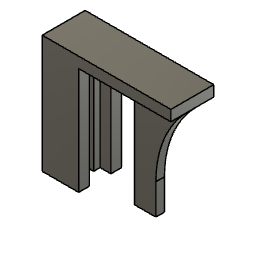
wall holder_ (Autodesk Fusion 360 design; units mm, degrees)
Autodesk Fusion 360 part; units mm, degrees
sketch "Esquisse1" plane through (0, 0, 0) normal (0, 1, 0) x (1, 0, 0)
  line L0 (-427, 120) -> (-367, 120)
  line L1 (-367, 120) -> (-367, 100)
  line L2 (-367, 100) -> (-427, 100)
  line L3 (-427, 100) -> (-427, 120)
  line L4 (-410, 120) -> (-410, 115)
  line L5 (-410, 115) -> (-415, 115)
  line L6 (-415, 115) -> (-415, 112)
  line L7 (-415, 112) -> (-417, 112)
  line L8 (-417, 112) -> (-417, 108)
  line L9 (-417, 108) -> (-415, 108)
  line L10 (-415, 105) -> (-415, 108)
  line L11 (-415, 105) -> (-410, 105)
  line L12 (-410, 100) -> (-410, 105)
  line L13 (-392, 112) -> (-382, 112)
  line L14 (-382, 112) -> (-382, 108)
  line L15 (-382, 108) -> (-392, 108)
  line L16 (-392, 108) -> (-392, 112)
  dimension "d5" = 20
  dimension "d6" = 60
  dimension "d7" = 5
  dimension "d8" = 3
  dimension "d9" = 5
  dimension "d10" = 2
  dimension "d12" = 4
  dimension "d13" = 3
  dimension "d14" = 2
  dimension "d15" = 5
  dimension "d16" = 5
  dimension "d17" = 10
  dimension "d18" = 4
  dimension "d19" = 25
  dimension "d26" = 10
  constraint horizontal L0
  constraint vertical L1
  constraint horizontal L2
  constraint vertical L3
  constraint coincident L0 L4.start
  constraint perpendicular L0 L4
  constraint perpendicular L4 L5
  constraint perpendicular L5 L6
  constraint perpendicular L6 L7
  constraint perpendicular L7 L8
  constraint perpendicular L8 L9
  constraint perpendicular L9 L10
  constraint perpendicular L10 L11
  constraint coincident L2 L12.start
  constraint perpendicular L11 L12
  constraint horizontal L13
  constraint vertical L14
  constraint horizontal L15
  constraint vertical L16
  measures "d5" distance of L0.end L1.end
  measures "d6" distance of L0.start L0.end
  measures "d7" distance of L4.start L4.end
  measures "d8" distance of L5.end L6.end
  measures "d9" distance of L4.end L5.end
  measures "d10" distance of L6.end L7.end
  measures "d12" distance of L7.end L8.end
  measures "d13" distance of L9.end L10.start
  measures "d14" distance of L8.end L9.end
  measures "d15" distance of L10.start L11.end
  measures "d16" distance of L11.end L12.start
  measures "d17" distance of L13.start L13.end
  measures "d18" distance of L13.end L14.end
  measures "d19" distance of L8 L16
  measures "d26" distance of L3 L8
extrude "Extrusion1" add sketch "Esquisse1" along normal blind 5 contours L0 L2 L3 L4 L5 L6 L7 L8 L9 L10 L11 L12 | L0 L1 L2 L4 L5 L6 L7 L8 L9 L10 L11 L12 | L13 L14 L15 L16
extrude "Extrusion2" add sketch "Esquisse1" against normal blind 50 contours L0 L2 L3 L4 L5 L6 L7 L8 L9 L10 L11 L12 | L13 L14 L15 L16
fillet "Congé1" radius 50 1 edges at (-382, 0, -110)
sketch "Esquisse2" plane through (0, 0, 0) normal (0, -1, 0) x (1, 0, 0)
  line L0 (-392, -108) -> (-367, -108)
  line L1 (-367, -108) -> (-367, -100)
  line L2 (-367, -100) -> (-410, -100)
  line L3 (-410, -100) -> (-410, -105)
  line L4 (-410, -105) -> (-415, -105)
  line L5 (-415, -105) -> (-415, -108)
  line L6 (-415, -108) -> (-417, -108)
  line L7 (-417, -108) -> (-417, -112)
  line L8 (-417, -112) -> (-415, -112)
  line L9 (-415, -112) -> (-415, -115)
  line L10 (-415, -115) -> (-410, -115)
  line L11 (-410, -115) -> (-410, -120)
  line L12 (-410, -120) -> (-367, -120)
  line L13 (-367, -120) -> (-367, -112)
  line L14 (-367, -112) -> (-392, -112)
  line L15 (-392, -112) -> (-392, -108)
  line L16 (-392, -112) -> (-417, -112)
  line L17 (-417, -112) -> (-417, -108)
  line L18 (-417, -108) -> (-392, -108)
  line L19 (-392, -108) -> (-392, -112)
  constraint horizontal L16
  constraint vertical L17
  constraint horizontal L18
  constraint vertical L19
  constraint coincident L6.end L7.start
  constraint coincident L14.end L15.start
extrude "Extrusion3" add sketch "Esquisse2" along normal blind 4 contours L6 L7 L8 L15 L16 L17 L18 L19
